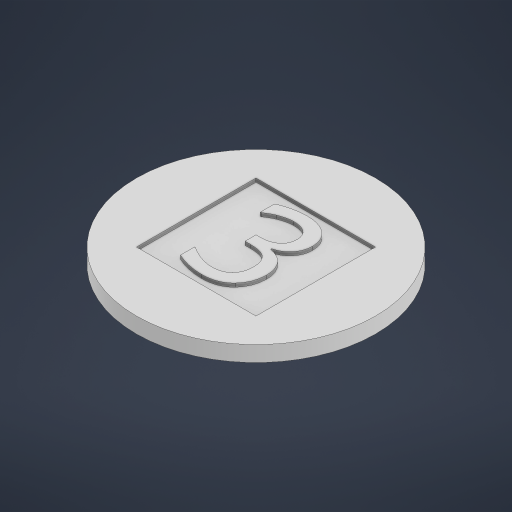
# Autodesk Inventor part: TopMarker3
Saved by Autodesk Inventor 2023 (Build 270158000, 158)
## iProperties
Created: 2023-03-04
Part Number: TopMarker3
Material: Generic
Document SubType Name: Modeling
Designer: Elias Braun
Density: 1 g/cm^3
Appearance: Default
Author: Elias Braun
Autodesk Inventor part; units mm, degrees
ref_plane "YZ Plane" through (0, 0, 0) normal (1, 0, 0) x (0, 1, 0)
ref_plane "XZ Plane" through (0, 0, 0) normal (0, 1, 0) x (-1, 0, 0)
ref_plane "XY Plane" through (0, 0, 0) normal (0, 0, 1) x (1, 0, 0)
sketch "Sketch1" plane through (0, 0, 0) normal (0, 1, 0) x (-1, 0, 0)
  circle A0 centre (0, 0) radius 20
  dimension "d0" = 40
  constraints: 1 centre point, 1 coincident
  measures "d0" diameter of A0
extrude "Extrusion1" add sketch "Sketch1" along normal blind 2.6
sketch "Sketch2" plane through (0, 2.6, 0) normal (0, 1, 0) x (1, 0, 0)
  line L0 (-10, -10) -> (-10, 10)
  line L1 (-10, 10) -> (10, 10)
  line L2 (10, 10) -> (10, -10)
  line L3 (10, -10) -> (-10, -10)
  line L4 (-10, -10) -> (10, 10) construction
  line L5 (-10, 10) -> (10, -10) construction
  point P0 (0, 0)
  dimension "d3" = 20
  dimension "d4" = 20
  constraints: 12 end point, 2 midpoint, 2 parallel, 1 perpendicular, 1 vertical
  measures "d3" distance of L0.start L0.end
  measures "d4" distance of L0.end L1.end
extrude "Extrusion2" cut sketch "Sketch2" against normal blind 0.6
sketch "Sketch3" plane through (0, 2, 0) normal (0, 1, 0) x (1, 0, 0)
  line L0 (-6.2284, 8.788) -> (6.2284, 8.788) construction
  line L1 (6.2284, 8.788) -> (6.2284, -8.5115) construction
  line L2 (6.2284, -8.5115) -> (-6.2284, -8.5115) construction
  line L3 (-6.2284, -8.5115) -> (-6.2284, 8.788) construction
  spline S0 degree 2 poles (-0.5381, 6.8643) (-1.1434, 6.8643) (-2.3407, 6.5684) (-2.9191, 6.3397) knots 0 0 0 1 2 2 2
  spline S1 degree 2 poles (-2.9191, 6.3397) (-3.4572, 6.111) (-4.2509, 5.6267) (-4.5603, 5.4115) knots 0 0 0 1 2 2 2
  line L4 (-4.5603, 5.4115) -> (-4.6948, 5.4115)
  line L5 (-4.6948, 5.4115) -> (-4.6948, 7.7656)
  spline S2 degree 2 poles (-4.6948, 7.7656) (-3.9684, 8.1557) (-1.4797, 8.788) (-0.3632, 8.788) knots 0 0 0 1 2 2 2
  spline S3 degree 2 poles (-0.3632, 8.788) (0.7668, 8.788) (2.4483, 8.3306) (3.1344, 7.8463) knots 0 0 0 1 2 2 2
  spline S4 degree 2 poles (3.1344, 7.8463) (3.8608, 7.3217) (4.6141, 5.8016) (4.6141, 4.7792) knots 0 0 0 1 2 2 2
  spline S5 degree 2 poles (4.6141, 4.7792) (4.6141, 3.4071) (2.8115, 1.3355) (1.547, 1.0664) knots 0 0 0 1 2 2 2
  line L6 (1.547, 1.0664) -> (1.547, 0.905)
  spline S6 degree 2 poles (1.547, 0.905) (2.0716, 0.7974) (3.2689, 0.3131) (3.7801, -0.1712) knots 0 0 0 1 2 2 2
  spline S7 degree 2 poles (3.7801, -0.1712) (4.2912, -0.642) (4.937, -2.1487) (4.937, -3.2383) knots 0 0 0 1 2 2 2
  spline S8 degree 2 poles (4.937, -3.2383) (4.937, -4.3548) (4.1702, -6.2516) (3.4707, -6.978) knots 0 0 0 1 2 2 2
  spline S9 degree 2 poles (3.4707, -6.978) (2.7442, -7.7313) (0.6861, -8.5115) (-0.6188, -8.5115) knots 0 0 0 1 2 2 2
  spline S10 degree 2 poles (-0.6188, -8.5115) (-1.8699, -8.5115) (-4.3182, -7.9062) (-5.1522, -7.4892) knots 0 0 0 1 2 2 2
  line L7 (-5.1522, -7.4892) -> (-5.1522, -5.135)
  line L8 (-5.1522, -5.135) -> (-4.9908, -5.135)
  spline S11 degree 2 poles (-4.9908, -5.135) (-4.2912, -5.6462) (-1.9237, -6.5879) (-0.7533, -6.5879) knots 0 0 0 1 2 2 2
  spline S12 degree 2 poles (-0.7533, -6.5879) (-0.0673, -6.5879) (1.3049, -6.1574) (1.7622, -5.6597) knots 0 0 0 1 2 2 2
  spline S13 degree 2 poles (1.7622, -5.6597) (2.2062, -5.162) (2.677, -3.9782) (2.677, -3.0769) knots 0 0 0 1 2 2 2
  spline S14 degree 2 poles (2.677, -3.0769) (2.677, -2.1756) (2.1524, -1.0052) (1.6815, -0.6689) knots 0 0 0 1 2 2 2
  spline S15 degree 2 poles (1.6815, -0.6689) (1.2107, -0.3326) (-0.0673, -0.077) (-0.8206, -0.077) knots 0 0 0 1 2 2 2
  line L9 (-0.8206, -0.077) -> (-1.7622, -0.077)
  line L10 (-1.7622, -0.077) -> (-1.7622, 1.7659)
  line L11 (-1.7622, 1.7659) -> (-1.0224, 1.7659)
  spline S16 degree 2 poles (-1.0224, 1.7659) (0.4708, 1.7659) (2.3541, 3.1919) (2.3541, 4.5505) knots 0 0 0 1 2 2 2
  spline S17 degree 2 poles (2.3541, 4.5505) (2.3541, 5.1828) (1.8699, 6.0841) (1.4797, 6.3531) knots 0 0 0 1 2 2 2
  spline S18 degree 2 poles (1.4797, 6.3531) (1.0627, 6.6356) (0.0404, 6.8643) (-0.5381, 6.8643) knots 0 0 0 1 2 2 2
  point P0 (0, 0)
  constraints: 2 other
extrude "Extrusion3" add sketch "Sketch3" along normal blind 0.6
body "Solid1"
